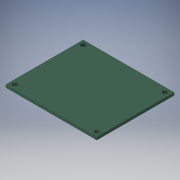
# Autodesk Inventor part: SparkFun GPS-RTK Dead Reckoning Breakout
Saved by Autodesk Inventor 2019 (Build 230136000, 136)
## iProperties
Created: 2020-08-03
Part Number: SparkFun GPS-RTK Dead Reckoning Breakout
Material: Generic
Document SubType Name: Modeling
Designer: james
Density: 1 g/cm^3
Appearance: Default(1)
Author: james
Autodesk Inventor part; units mm, degrees
ref_plane "YZ Plane" through (0, 0, 0) normal (1, 0, 0) x (0, 1, 0)
ref_plane "XZ Plane" through (0, 0, 0) normal (0, 1, 0) x (-1, 0, 0)
ref_plane "XY Plane" through (0, 0, 0) normal (0, 0, 1) x (1, 0, 0)
sketch "Sketch1" plane through (0, 0, 0) normal (0, 1, 0) x (-1, 0, 0)
  line L0 (30.1019, 31.2653) -> (-20.6981, 31.2653)
  line L1 (-20.6981, 31.2653) -> (-20.6981, -11.9147)
  line L2 (-20.6981, -11.9147) -> (30.1019, -11.9147)
  line L3 (30.1019, -11.9147) -> (30.1019, 31.2653)
  point P0 (0, 0)
  dimension "d0" = 50.8
  dimension "d1" = 43.18
  constraints: 8 end point, 2 parallel, 1 horizontal, 1 perpendicular
  measures "d0" distance of L0.start L0.end
  measures "d1" distance of L2.end L0.start
extrude "Extrusion1" add sketch "Sketch1" along normal blind 1.524
sketch "Sketch2" plane through (0, 1.524, 0) normal (0, 1, 0) x (1, 0, 0)
  line L0 (20.6981, -31.2653) -> (20.6981, 11.9147) projected
  line L1 (-30.1019, -31.2653) -> (20.6981, -31.2653) projected
  line L2 (20.6981, 11.9147) -> (-30.1019, 11.9147) projected
  line L3 (-30.1019, 11.9147) -> (-30.1019, -31.2653) projected
  point P0 (0, 0)
  point P1 (-27.5619, -28.7253)
  point P2 (-27.5619, 9.3747)
  point P3 (18.1581, 9.3747)
  point P4 (18.1581, -28.7253)
  dimension "d4" = 0
  dimension "d5" = 0
  dimension "d6" = 0
  dimension "d7" = 0
  dimension "d8" = 2.54
  dimension "d9" = 2.54
  dimension "d10" = 2.54
  dimension "d18" = 2.54
  measures "d4" vertical distance of point (18.158, -28.725) point (-27.562, -28.725)
  measures "d5" vertical distance of point (18.158, 9.375) point (-27.562, 9.375)
  measures "d6" horizontal distance of point (-27.562, -28.725) point (-27.562, 9.375)
  measures "d7" horizontal distance of point (18.158, 9.375) point (18.158, -28.725)
  measures "d8" distance from line of L0 point (18.158, 9.375)
  measures "d9" distance from line of L1 point (18.158, -28.725)
  measures "d10" distance from line of L2 point (-27.562, 9.375)
  measures "d18" distance from line of L3 point (-27.562, 9.375)
hole "Hole1" at (-27.5619, 1.524, 28.7253) at (-27.5619, 1.524, -9.3747) at (18.1581, 1.524, -9.3747) at (18.1581, 1.524, 28.7253) direction (0, -1, 0) diameter 2.4638 end through all
body "Solid1"
